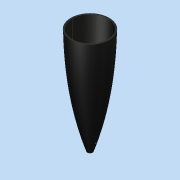
# Autodesk Inventor part: PrimarySingleAft_03
Saved by Autodesk Inventor 2017 (Build 210142000, 142)
## iProperties
Created: 2016-09-09
Part Number: PrimarySingleAft_03
Material: Generic
Document SubType Name: Modeling
Designer: techn
Density: 1 g/cm^3
Appearance: Glossy - Black
Mass: 1301.69 g
Surface Area: 728.736 cm^2
Volume: 1301.69 cm^3
Author: techn
Autodesk Inventor part; units mm, degrees
ref_plane "YZ Plane" through (0, 0, 0) normal (1, 0, 0) x (0, 1, 0)
ref_plane "XZ Plane" through (0, 0, 0) normal (0, 1, 0) x (-1, 0, 0)
ref_plane "XY Plane" through (0, 0, 0) normal (0, 0, 1) x (1, 0, 0)
sketch "Sketch2" plane through (0, 0, 0) normal (0, 0, 1) x (1, 0, 0)
  line L0 (-528.9365, -48.3632) -> (-528.9365, 1201.5435) construction
  line L1 (-528.9365, 1201.5435) -> (398.4136, 1201.5435) construction
  line L2 (398.4136, 1201.5435) -> (398.4136, -48.3632) construction
  line L3 (398.4136, -48.3632) -> (-528.9365, -48.3632) construction
  point P0 (0, 0)
  constraints: 2 other
sketch "Sketch1" plane through (0, 0, 0) normal (0, 0, 1) x (1, 0, 0)
  line L0 (0, 0) -> (0, 299.212)
  line L1 (0, 299.212) -> (50.8, 299.212)
  line L2 (50.8, 299.212) -> (-50.8, 299.212)
  line L3 (-50.8, 299.212) -> (-43.9085, -128.4284) construction
  line L4 (-43.9085, -128.4284) -> (249.7404, -308.1211) construction
  spline S0 degree 2 poles (-50.8, 299.212) (-43.9085, -128.4284) (249.7404, -308.1211) knots 1 1 1 2 2 2
  line L5 (50.8, 299.212) -> (43.9085, -128.4284) construction
  line L6 (43.9085, -128.4284) -> (-249.7404, -308.1211) construction
  spline S1 degree 2 poles (50.8, 299.212) (43.9085, -128.4284) (-249.7404, -308.1211) knots 1 1 1 2 2 2
  line L7 (-6.945, 18.1993) -> (0, 18.1993)
  line L8 (0, 18.1993) -> (0, 299.212)
  line L9 (0, 299.212) -> (-50.8, 299.212)
  dimension "d0" = 299.212
  dimension "d1" = 50.8
  dimension "d2" = 101.6
  dimension "d50" = 281.0127
  constraints: 12 end point, 3 perpendicular, 2 point on line, 2 symmetric about line, 1 collinear, 1 vertical, 7 other
  measures "d0" distance of L0.start L0.end
  measures "d1" distance of L0.end L1.end
  measures "d2" distance of L1.end L2.end
  measures "d50" distance between parallel lines of L2 L7
revolve "Revolution1" add sketch "Sketch1" angle 360 about axis through (0, 0, 0) along (0, 1, 0) contours L7 S0 L2 L0
shell "Shell1" thickness 3.175 removed faces 1 at (-11.9737, 299.212, 11.9737)
sketch "Sketch3" plane through (0, 0, 0) normal (0, 0, 1) x (1, 0, 0)
  line L0 (6.945, 18.1993) -> (-6.945, 18.1993) projected
  line L1 (50.8, 299.212) -> (-50.8, 299.212) projected
  line L2 (0, 18.1993) -> (0, 43.5993)
  line L3 (23.4579, 43.5993) -> (-26.0828, 43.5993)
  line L4 (-26.0828, 43.5993) -> (-26.0828, 45.1868)
  line L5 (-26.0828, 45.1868) -> (23.4579, 45.1868)
  line L6 (23.4579, 45.1868) -> (23.4579, 43.5993)
  point P0 (0, 0)
  dimension "d40" = 25.4
  dimension "d41" = 1.5875
  constraints: 10 end point, 2 parallel, 1 horizontal, 1 midpoint, 1 perpendicular, 1 vertical, 1 other
  measures "d40" distance of L2.start L2.end
  measures "d41" distance of L3.end L4.end
revolve "Revolution2" cut sketch "Sketch3" angle 360 about axis through (23.4579, 43.5993, 0) along (-1, 0, 0)
sketch "Sketch4" plane through (0, 18.1993, 0) normal (0, -1, 0) x (1, 0, 0)
  circle A0 centre (0, 0) radius 6.945 projected
  circle A1 centre (0, 0) radius 3.175
  point P0 (-6.945, 0)
  dimension "d43" = 6.35
  constraints: 1 centre point, 1 coincident, 1 horizontal alignment
  measures "d43" diameter of A1
extrude "Extrusion1" cut sketch "Sketch4" against normal up to surface (3.175 mm away) contours A1
sketch "Sketch7" plane through (0, 0, 0) normal (0, 0, 1) x (1, 0, 0)
  line L0 (-3.175, 21.3743) -> (3.175, 21.3743) projected
  line L1 (3.175, 21.3743) -> (6.35, 21.3743)
  line L2 (6.35, 21.3743) -> (6.35, 24.5493)
  line L3 (6.35, 24.5493) -> (3.175, 24.5493)
  line L4 (3.175, 24.5493) -> (3.175, 21.3743)
  line L5 (0, 21.3743) -> (0, 23.4701)
  line L6 (0, 23.4701) -> (0, 15.284)
  point P0 (0, 0)
  dimension "d46" = 3.175
  dimension "d47" = 3.175
  constraints: 12 end point, 2 parallel, 1 horizontal, 1 midpoint, 1 perpendicular, 1 point on line, 1 vertical
  measures "d46" distance of L3.end L2.end
  measures "d47" distance of L2.end L1.end
revolve "Revolution3" add sketch "Sketch7" angle 360 about axis through (0, 23.4701, 0) along (0, -1, 0)
body "Solid1"
